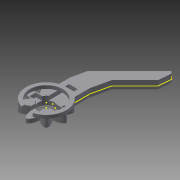
# Autodesk Inventor part: BrazoPinza2
Saved by Autodesk Inventor 2015 (Build 190159000, 159)
## iProperties
Created: 2013-11-10
Part Number: BrazoPinza2
Material: Genérico
Document SubType Name: Modeling
Designer: Gregorio
Density: 1 g/cm^3
Appearance: Valor por defecto
Author: Gregorio
Autodesk Inventor part; units mm, degrees
ref_plane "YZ Plane" through (0, 0, 0) normal (1, 0, 0) x (0, 1, 0)
ref_plane "XZ Plane" through (0, 0, 0) normal (0, 1, 0) x (-1, 0, 0)
ref_plane "XY Plane" through (0, 0, 0) normal (0, 0, 1) x (1, 0, 0)
sketch "Boceto1" plane through (0, 0, 0) normal (0, 0, 1) x (1, 0, 0)
  circle A0 centre (0, 0) radius 12.5
  circle A1 centre (0, 0) radius 4
  ellipse E0 centre (0, 4) end of major axis (0, 12.5) minor radius 3
  ellipse E1 centre (2.85, 2.806688) end of major axis (8.917459, 8.759504) minor radius 3
  ellipse E2 centre (4, 0) end of major axis (12.5, 0) minor radius 3
  ellipse E3 centre (2.85, -2.806688) end of major axis (8.803082, -8.874419) minor radius 3
  ellipse E4 centre (0, -4) end of major axis (0, -12.5) minor radius 3
  ellipse E5 centre (-2.85, -2.806688) end of major axis (-8.917459, -8.759504) minor radius 3
  ellipse E6 centre (-4, 0) end of major axis (-12.5, 0) minor radius 3
  ellipse E7 centre (-2.85, 2.806688) end of major axis (-8.803082, 8.874419) minor radius 3
  dimension "d1" = 8
  dimension "d4" = 3
  dimension "d5" = 3
  dimension "d6" = 3
  dimension "d7" = 3
  dimension "d8" = 3
  dimension "d9" = 3
  dimension "d10" = 3
  dimension "d11" = 3
  dimension "d0" = 25
  dimension "d12" = 2.85
  dimension "d14" = 2.85
  dimension "d15" = 2.85
  dimension "d16" = 2.85
  constraints: 2 coincident, 2 horizontal alignment, 2 vertical alignment, 1 centre point, 34 other
  measures "d0" diameter of A0
  measures "d12" horizontal distance of point (2.85, 2.807) point (0, 4)
  measures "d14" horizontal distance of point (-2.85, 2.807) point (0, 4)
  measures "d15" horizontal distance of point (0, -4) point (-2.85, -2.807)
  measures "d16" horizontal distance of point (2.85, -2.807) point (0, -4)
sketch "Boceto1 outline for Extrusión1" plane through (0, 0, 0) normal (0, 0, 1) x (1, 0, 0)
  spline S0 degree 2 poles (6.837651, -2.827888) (12.5, -2.120108) (12.5, 0) knots 0 0 0 1 1 1 weights 1 0.8166521 1
  spline S1 degree 2 poles (12.5, 0) (12.5, 2.10484) (6.892108, 2.821007) knots 0 0 0 1 1 1 weights 1 0.81861101 1
  spline S2 degree 2 poles (6.892108, 2.821007) (10.390906, 7.257681) (8.917459, 8.759504) knots 0 0 0 1 1 1 weights 1 0.81872774 1
  spline S3 degree 2 poles (8.917459, 8.759504) (7.418259, 10.287577) (2.836507, 6.767727) knots 0 0 0 1 1 1 weights 1 0.81400986 1
  spline S4 degree 2 poles (2.836507, 6.767727) (2.139767, 12.5) (0, 12.5) knots 0 0 0 1 1 1 weights 1 0.81412987 1
  spline S5 degree 2 poles (0, 12.5) (-2.124614, 12.5) (-2.829887, 6.821604) knots 0 0 0 1 1 1 weights 1 0.81607395 1
  spline S6 degree 2 poles (-2.829887, 6.821604) (-7.292525, 10.356434) (-8.803082, 8.874419) knots 0 0 0 1 1 1 weights 1 0.81715812 1
  spline S7 degree 2 poles (-8.803082, 8.874419) (-10.322463, 7.383746) (-6.837651, 2.827888) knots 0 0 0 1 1 1 weights 1 0.81557201 1
  spline S8 degree 2 poles (-6.837651, 2.827888) (-12.5, 2.120108) (-12.5, 0) knots 0 0 0 1 1 1 weights 1 0.8166521 1
  spline S9 degree 2 poles (-12.5, 0) (-12.5, -2.10484) (-6.892108, -2.821007) knots 0 0 0 1 1 1 weights 1 0.81861101 1
  spline S10 degree 2 poles (-6.892108, -2.821007) (-10.390906, -7.257681) (-8.917459, -8.759504) knots 0 0 0 1 1 1 weights 1 0.81872774 1
  spline S11 degree 2 poles (-8.917459, -8.759504) (-7.418259, -10.287577) (-2.836507, -6.767727) knots 0 0 0 1 1 1 weights 1 0.81400986 1
  spline S12 degree 2 poles (-2.836507, -6.767727) (-2.139767, -12.5) (0, -12.5) knots 0 0 0 1 1 1 weights 1 0.81412987 1
  spline S13 degree 2 poles (0, -12.5) (2.124614, -12.5) (2.829887, -6.821604) knots 0 0 0 1 1 1 weights 1 0.81607395 1
  spline S14 degree 2 poles (2.829887, -6.821604) (7.292525, -10.356434) (8.803082, -8.874419) knots 0 0 0 1 1 1 weights 1 0.81715812 1
  spline S15 degree 2 poles (8.803082, -8.874419) (10.322463, -7.383746) (6.837651, -2.827888) knots 0 0 0 1 1 1 weights 1 0.81557201 1
extrude "Extrusión1" add sketch "Boceto1 outline for Extrusión1" along normal blind 2
sketch "Boceto8" plane through (0, 0, 2) normal (0, 0, 1) x (1, 0, 0)
  ellipse E0 centre (0, -4) end of major axis (0, 4.5) minor radius 3 (-2.836507, -6.767727) -> (2.829887, -6.821604) ccw
  line L0 (-6, 0) -> (6, 0)
  line L1 (6, 0) -> (6, 30)
  line L2 (6, 30) -> (-6, 30)
  line L3 (-6, 30) -> (-6, 0)
  point P0 (-0.999598, -4.241115)
  point P1 (0.999598, -4.241115)
  point P2 (3.724042, 2.263875)
  point P3 (2.320169, 3.687234)
  point P4 (-2.322293, 3.696019)
  point P5 (-3.715493, 2.261418)
  dimension "d42" = 30
  constraints: 8 end point, 2 parallel, 1 horizontal, 1 perpendicular, 1 other
  measures "d42" distance of L1.end L0.end
extrude "Extrusión7" add sketch "Boceto8" along normal blind 3
sketch "Boceto3" plane through (0, 0, 2) normal (0, 0, 1) x (1, 0, 0)
  circle A0 centre (0, 0) radius 5
  dimension "d19" = 10
  constraints: 1 centre point
  measures "d19" diameter of A0
extrude "Extrusión2" cut sketch "Boceto3" along normal mid plane 10
sketch "Boceto23" plane through (0, 0, 2) normal (0, 0, 1) x (1, 0, 0)
  arc A0 (-5, 0) -> (5, 0) centre (0, 0) ccw
  line L0 (-5, 0) -> (-6, 0)
  line L1 (-6, 0) -> (-6, 8.791069)
  ellipse E0 centre (-2.85, 2.806688) end of major axis (3.103082, -3.261042) minor radius 3 (-6, 8.791069) -> (-6.837651, 2.827888) ccw
  ellipse E1 centre (-4, 0) end of major axis (4.5, 0) minor radius 3 (-6.837651, 2.827888) -> (-6.892108, -2.821007) ccw
  ellipse E2 centre (-2.85, -2.806688) end of major axis (3.217459, 3.146128) minor radius 3 (-6.892108, -2.821007) -> (-2.836507, -6.767727) ccw
  ellipse E3 centre (0, -4) end of major axis (0, 4.5) minor radius 3 (-2.836507, -6.767727) -> (2.829887, -6.821604) ccw
  ellipse E4 centre (2.85, -2.806688) end of major axis (-3.103082, 3.261042) minor radius 3 (2.829887, -6.821604) -> (6.837651, -2.827888) ccw
  ellipse E5 centre (4, 0) end of major axis (-4.5, 0) minor radius 3 (6.837651, -2.827888) -> (6.892108, 2.821007) ccw
  ellipse E6 centre (2.85, 2.806688) end of major axis (-3.217459, -3.146128) minor radius 3 (6.892108, 2.821007) -> (6, 8.683177) ccw
  line L2 (6, 8.683177) -> (6, 0)
  line L3 (6, 0) -> (5, 0)
  constraints: 7 other
sketch "Boceto23 outline for Extrusión20" plane through (0, 0, 2) normal (0, 0, 1) x (1, 0, 0)
  line L0 (6, 0) -> (5, 0)
  line L1 (6, 8.683177) -> (6, 0)
  spline S0 degree 2 poles (6.892108, 2.821007) (14.233977, 12.130911) (6, 8.683177) knots 0 0 0 1 1 1 weights 1 0.56203853 1
  spline S1 degree 2 poles (6.837651, -2.827888) (29.218919, -0.030284) (6.892108, 2.821007) knots 0 0 0 1 1 1 weights 1 0.33704659 1
  spline S2 degree 2 poles (2.829887, -6.821604) (20.749751, -21.015825) (6.837651, -2.827888) knots 0 0 0 1 1 1 weights 1 0.33290635 1
  spline S3 degree 2 poles (-2.836507, -6.767727) (-0.03062, -29.852537) (2.829887, -6.821604) knots 0 0 0 1 1 1 weights 1 0.328786 1
  spline S4 degree 2 poles (-6.892108, -2.821007) (-21.021817, -20.738274) (-2.836507, -6.767727) knots 0 0 0 1 1 1 weights 1 0.33293827 1
  spline S5 degree 2 poles (-6.837651, 2.827888) (-29.218919, 0.030284) (-6.892108, -2.821007) knots 0 0 0 1 1 1 weights 1 0.33704659 1
  spline S6 degree 2 poles (-6, 8.791069) (-13.992867, 12.182235) (-6.837651, 2.827888) knots 0 0 0 1 1 1 weights 1 0.56593193 1
  line L2 (-6, 0) -> (-6, 8.791069)
  line L3 (-5, 0) -> (-6, 0)
  arc A0 (5, 0) -> (-5, 0) centre (0, 0) cw
extrude "Extrusión20" add sketch "Boceto23 outline for Extrusión20" along normal blind 3
sketch "Boceto14" plane through (0, 0, 5) normal (0, 0, 1) x (1, 0, 0)
  circle A0 centre (0, 0) radius 5 projected
  line L0 (-2.75, -17) -> (2.75, -17)
  line L1 (2.75, -17) -> (2.75, 17)
  line L2 (2.75, 17) -> (-2.75, 17)
  line L3 (-2.75, 17) -> (-2.75, -17)
  line L4 (-2.75, -17) -> (2.75, 17) construction
  line L5 (2.75, -17) -> (-2.75, 17) construction
  line L6 (-8.5, 2) -> (8.5, 2)
  line L7 (8.5, 2) -> (8.5, -2)
  line L8 (8.5, -2) -> (-8.5, -2)
  line L9 (-8.5, -2) -> (-8.5, 2)
  line L10 (-8.5, 2) -> (8.5, -2) construction
  line L11 (8.5, 2) -> (-8.5, -2) construction
  dimension "d45" = 5.5
  dimension "d46" = 34
  dimension "d47" = 17
  dimension "d48" = 4
  constraints: 24 end point, 4 midpoint, 4 parallel, 2 horizontal, 2 perpendicular
  measures "d45" distance of L2.end L1.end
  measures "d46" distance of L1.end L0.end
  measures "d47" distance of L7.end L8.end
  measures "d48" distance of L6.end L7.end
extrude "Extrusión12" cut sketch "Boceto14" against normal blind 2.5 contours A0 L8 L1 L6 | A0 L6 L7 L8 | A0 L3 L2 L1 | L1 L8 L3 L6 | L1 L0 L3 A0 | L3 L8 A0 L6 | A0 L8 L9 L6
sketch "Boceto24" plane through (0, 0, 5) normal (0, 0, 1) x (1, 0, 0)
  line L0 (6, 30) -> (1, 35)
  line L1 (1, 35) -> (22.213203, 56.213203)
  line L2 (22.213203, 56.213203) -> (27.213203, 51.213203)
  line L3 (27.213203, 51.213203) -> (6, 30)
  line L4 (6, 30) -> (-6, 30)
  dimension "d80" = 30
  dimension "d81" = 5
  dimension "d92" = 45
  constraints: 8 end point, 2 parallel, 1 perpendicular
  measures "d80" distance of L0.end L1.end
  measures "d81" horizontal distance of L0.start L0.end
  measures "d92" angle of L4 L0
extrude "Extrusión21" add sketch "Boceto24" against normal blind 3
sketch "Boceto26" plane through (1, 35, 5) normal (-0.7071068, -0.7071068, 0) x (-0.7071068, 0.7071068, 0)
  line L0 (0, 0) -> (-7.071068, 0)
  line L1 (0, 0) -> (0, 3)
  line L2 (-7.071068, 3) -> (0, 3)
  line L3 (-7.071068, 3) -> (-7.071068, 0)
  point P0 (-24.041631, 5)
extrude "Extrusión23" add sketch "Boceto26" along normal up to next
sketch "Boceto27" plane through (0, 0, 5) normal (0, 0, 1) x (1, 0, 0)
  line L0 (-4, 30) -> (-5.952374, 21.214316)
  line L1 (-5.952374, 21.214316) -> (-13.046492, 22.790787)
  line L2 (-13.046492, 22.790787) -> (-11.094118, 31.576471)
  line L3 (-11.094118, 31.576471) -> (-4, 30)
  dimension "d94" = 9
  constraints: 8 end point, 2 parallel, 1 perpendicular
  measures "d94" distance of L1.end L2.end
extrude "Extrusión24" cut sketch "Boceto27" against normal blind 3
sketch "Boceto28" plane through (0, 0, 5) normal (0, 0, 1) x (1, 0, 0)
  line L0 (-4, 30) -> (-5.952374, 21.214316)
  line L1 (6, 8.683177) -> (6, 30)
  line L2 (6, 30) -> (27.213203, 51.213203)
  line L3 (6, 21.25) -> (8.5, 32.5)
  line L4 (8.5, 32.5) -> (5.058824, 33.264706)
  line L5 (5.058824, 33.264706) -> (2.558824, 22.014706)
  line L6 (2.558824, 22.014706) -> (6, 21.25)
  point P0 (-6, 21)
  dimension "d95" = 2.5
  constraints: 8 end point, 3 parallel, 2 point on line, 1 perpendicular
  measures "d95" horizontal distance of L3.end L1.end
extrude "Extrusión25" add sketch "Boceto28" against normal blind 3 contours L1 L2 L3
chamfer "Chaflán5" distance 5 angle 50 1 edges at (27.2132, 51.2132, 3.5) measured on face at (25.5465, 52.8799, 4)
sketch "Boceto29" plane through (0, 0, 5) normal (0, 0, 1) x (1, 0, 0)
  arc A0 (4.582576, 2) -> (2.75, 4.175823) centre (0, 0) ccw
  circle A1 centre (0, 0) radius 12.601536
  circle A2 centre (0, 0) radius 10.285357
  constraints: 2 centre point, 2 coincident
extrude "Extrusión26" add sketch "Boceto29" along normal blind 2
sketch "Boceto30" plane through (0, 0, 7) normal (0, 0, 1) x (1, 0, 0)
  circle A0 centre (0, 0) radius 10.285357
  line L0 (-3.5, 0) -> (3.5, 0)
  line L1 (3.5, 0) -> (3.5, -17)
  line L2 (3.5, -17) -> (-3.5, -17)
  line L3 (-3.5, -17) -> (-3.5, 0)
  point P0 (0, 0)
  dimension "d101" = 7
  constraints: 8 end point, 2 parallel, 1 coincident, 1 horizontal, 1 midpoint, 1 perpendicular
  measures "d101" distance of L1.end L2.end
extrude "Extrusión27" cut sketch "Boceto30" against normal blind 2 contours L3 L0 L1 A0 | A0 L1 L2 L3 picked at (0.395929, -3.405514)
sketch "Boceto31" plane through (0, 0, 2) normal (0, 0, -1) x (-1, 0, 0)
  line L0 (-22.999718, 46.999718) -> (-23.67767, 54.748737)
  line L1 (-22.999718, 46.999718) -> (-8.5, 32.5)
  line L2 (-8.5, 32.5) -> (-6, 21.25)
  line L3 (-6, 8.683177) -> (-6, 21.25)
  ellipse E0 centre (-2.85, 2.806688) end of major axis (3.217459, -3.146128) minor radius 3 (-2.836507, 6.767727) -> (-6, 8.683177) ccw
  ellipse E1 centre (0, 4) end of major axis (0, -4.5) minor radius 3 (2.829887, 6.821604) -> (-2.836507, 6.767727) ccw
  ellipse E2 centre (2.85, 2.806688) end of major axis (-3.103082, -3.261042) minor radius 3 (6, 8.791069) -> (2.829887, 6.821604) ccw
  line L4 (6, 21.2249) -> (6, 8.791069)
  line L5 (6, 21.2249) -> (5.952374, 21.214316)
  line L6 (5.952374, 21.214316) -> (4, 30)
  line L7 (-22.213203, 56.213203) -> (4, 30)
  line L8 (-22.213203, 56.213203) -> (-23.67767, 54.748737)
  point P0 (0, 0)
  constraints: 3 other
sketch "Boceto32" plane through (0, 0, 2) normal (0, 0, -1) x (-1, 0, 0)
  line L0 (-22.999718, 46.999718) -> (-23.67767, 54.748737)
  line L1 (-22.999718, 46.999718) -> (-8.5, 32.5)
  line L2 (-8.5, 32.5) -> (-6, 21.25)
  line L3 (-6, 8.683177) -> (-6, 21.25)
  ellipse E0 centre (-2.85, 2.806688) end of major axis (3.217459, -3.146128) minor radius 3 (-2.836507, 6.767727) -> (-6, 8.683177) ccw
  ellipse E1 centre (0, 4) end of major axis (0, -4.5) minor radius 3 (2.829887, 6.821604) -> (-2.836507, 6.767727) ccw
  ellipse E2 centre (2.85, 2.806688) end of major axis (-3.103082, -3.261042) minor radius 3 (6, 8.791069) -> (2.829887, 6.821604) ccw
  line L4 (6, 21.2249) -> (6, 8.791069)
  line L5 (6, 21.2249) -> (5.952374, 21.214316)
  line L6 (5.952374, 21.214316) -> (4, 30)
  line L7 (-22.213203, 56.213203) -> (4, 30)
  line L8 (-22.213203, 56.213203) -> (-23.67767, 54.748737)
  point P0 (0, 0)
  constraints: 3 other
extrude "Extrusión28" add sketch "Boceto31" along normal blind 2
